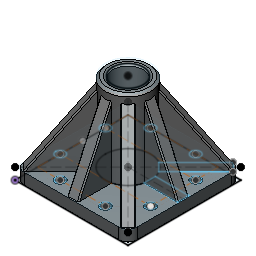
Кронштейн под лампу v1 (Autodesk Fusion 360 design; units mm, degrees)
Autodesk Fusion 360 part; units mm, degrees
sketch "Sketch1" plane through (0, 0, 0) normal (0, 0, 1) x (1, 0, 0)
  line L0 (0, 0) -> (50, 0)
  line L1 (50, 0) -> (50, 50)
  line L2 (50, 50) -> (0, 50)
  line L3 (0, 50) -> (0, 0)
  dimension "d1" = 50
  dimension "d2" = 50
  constraint horizontal L0
  constraint vertical L1
  constraint horizontal L2
  constraint vertical L3
  constraint coincident L0.start L3.end
  measures "d1" distance of L0.start L0.end
  measures "d2" distance of L0.start L2.end
extrude "Extrude1" add sketch "Sketch1" along normal blind 5 makes body 1
sketch "Sketch2" plane through (0, 0, 5) normal (0, 0, 1) x (-1, 0, 0)
  line L0 (0, -50) -> (0, 0)
  line L1 (0, 0) -> (-50, 0)
  line L2 (-50, 0) -> (-50, -50)
  line L3 (-50, -50) -> (0, -50)
  circle A0 centre (-25, -25) radius 10
  line L4 (0, -50) -> (-50, 0) construction
  line L5 (-50, -50) -> (0, 0) construction
  line L6 (-25, -25) -> (-50, -25) construction
  line L7 (-34.6825, -22.5) -> (-49.4483, -22.5)
  line L8 (-49.4483, -22.5) -> (-49.4483, -27.5)
  line L9 (-34.6825, -27.5) -> (-49.4483, -27.5)
  line L10 (-34.6825, -27.5) -> (-34.6825, -22.5)
  line L11 (-50, -46.4645) -> (-46.4645, -50)
  line L12 (-46.4645, -50) -> (-30.0788, -33.6143)
  line L13 (-30.0788, -33.6143) -> (-33.6143, -30.0788)
  line L14 (-33.6143, -30.0788) -> (-50, -46.4645)
  line L15 (-45, -35) -> (-45, -45) construction
  line L16 (-45, -45) -> (-35, -45) construction
  line L17 (-35, -45) -> (-25, -45) construction
  line L18 (-25, -45) -> (-15, -45) construction
  line L19 (-15, -45) -> (-5, -45) construction
  line L20 (-5, -45) -> (-5, -35) construction
  line L21 (-5, -35) -> (-45, -35) construction
  line L22 (-45, -35) -> (-45, -15) construction
  line L23 (-45, -15) -> (-5, -15) construction
  line L24 (-5, -15) -> (-5, -25) construction
  line L25 (-5, -15) -> (-5, -5) construction
  line L26 (-5, -5) -> (-15, -5) construction
  line L27 (-15, -5) -> (-35, -5) construction
  circle A1 centre (-45, -35) radius 2
  circle A2 centre (-45, -15) radius 2
  circle A3 centre (-5, -35) radius 2
  circle A4 centre (-35, -45) radius 2
  circle A5 centre (-15, -45) radius 2
  circle A6 centre (-5, -15) radius 2
  circle A7 centre (-15, -5) radius 2
  circle A8 centre (-35, -5) radius 2
  dimension "d5" = 20
  dimension "d18" = 5
  dimension "d32" = 10
  dimension "d33" = 10
  dimension "d34" = 10
  dimension "d35" = 10
  dimension "d36" = 4
  dimension "d43" = 4
  dimension "d44" = 4
  dimension "d45" = 4
  dimension "d46" = 4
  dimension "d47" = 4
  dimension "d48" = 4
  dimension "d49" = 4
  constraint coincident L0.start L3.end
  constraint coincident L1.end L2.start
  constraint coincident L2.end L3.start
  constraint coincident L0.end L1.start
  constraint midpoint A0.centre L5
  constraint coincident A0.centre L6.start
  constraint midpoint L2 L6.end
  constraint perpendicular L6 L8
  constraint coincident A0 L9.start
  constraint perpendicular L8 L9
  constraint coincident A0 L7.start
  constraint horizontal L7
  constraint coincident L2 L11.start
  constraint coincident L3 L11.end
  constraint coincident A0 L12.end
  constraint perpendicular L11 L12
  constraint coincident A0 L13.end
  constraint perpendicular L5 L13
  constraint perpendicular L11 L14
  constraint coincident L5 L15.end
  constraint vertical L15
  constraint perpendicular L15 L16
  constraint parallel L16 L17
  constraint parallel L17 L18
  constraint coincident L4 L19.end
  constraint perpendicular L0 L19
  constraint perpendicular L19 L20
  constraint perpendicular L15 L21
  constraint perpendicular L7 L22
  constraint perpendicular L22 L23
  constraint perpendicular L21 L24
  constraint perpendicular L23 L25
  constraint perpendicular L25 L26
  constraint perpendicular L25 L27
  constraint coincident L15.start L21.end
  constraint coincident L16.end L17.start
  constraint coincident L18.end L19.start
  constraint coincident L23.end L24.start
  constraint coincident L26.end L27.start
  constraint coincident L27.end A8.centre
  measures "d5" diameter of A0
  measures "d18" distance of L7.end L8.end
  measures "d32" distance of L15.end L16.end
  measures "d33" distance of L17.end L18.end
  measures "d34" distance of L23.end L25.end
  measures "d35" distance of L25.end L26.end
  measures "d36" diameter of A1
  measures "d43" diameter of A2
  measures "d44" diameter of A3
  measures "d45" diameter of A4
  measures "d46" diameter of A5
  measures "d47" diameter of A6
  measures "d48" diameter of A7
  measures "d49" diameter of A8
extrude "Extrude2" add sketch "Sketch2" along normal blind 35 contours A0 L10 L13 | A0 L13 | A0 L10 bodies 1
sketch "Sketch3" plane through (0, 0, 40) normal (0, 0, 1) x (-1, 0, 0)
  circle A0 centre (-25, -25) radius 10
  circle A1 centre (-25, -25) radius 6.75
  dimension "d8" = 13.5
  constraint concentric A0 A1
  measures "d8" diameter of A1
extrude "Extrude3" cut sketch "Sketch3" against normal blind 40 contours A1 bodies 1
extrude "Extrude4" add sketch "Sketch2" along normal blind 33 separate body contours A0 L7 L8 L9 makes body 2
extrude "Extrude5" add sketch "Sketch2" along normal blind 33 separate body contours A0 L11 L12 L14 makes body 3
draft "Draft1" angle 25 neutral plane through (0, 0, 5) pull (0, 0, 1) 1 faces at (49.4483, 24.1667, 16) on bodies 2
draft "Draft2" angle 36.3 neutral plane through (0, 0, 5) pull (0, 0, 1) 1 faces at (47.643, 48.8215, 27) on bodies 3
pattern_circular "C-Pattern1" count 4 over 360 about axis through (25, 25, 5) along (0, 0, 1) of bodies 2 makes body 4 at (22.5, 39.6044, 15.5552) makes body 5 at (10.3956, 22.5, 15.5552) makes body 6 at (27.5, 10.3956, 15.5552)
pattern_circular "C-Pattern2" count 4 over 360 about axis through (25, 25, 5) along (0, 0, 1) of bodies 3 makes body 7 at (14.4593, 39.0762, 15.5154) makes body 8 at (10.9238, 14.4593, 15.5154) makes body 9 at (35.5407, 10.9238, 15.5154)
extrude "Extrude9" cut sketch "Sketch2" against normal blind 5 contours A1 | A2 | A3 | A4 | A5 | A6 | A7 | A8 bodies 1
chamfer "Chamfer1" distance 1 angle 45 1 edges at (31.2932, 22.5591, 40) on bodies 1
chamfer "Chamfer2" distance 1 angle 45 1 edges at (34.3233, 28.6162, 40) on bodies 1
chamfer "Chamfer3" distance 0.5 angle 45 16 edges at (22.5, 42.0654, 20.8327) (27.5, 42.0654, 20.8327) (38.2716, 41.8071, 20.773) (41.8071, 38.2716, 20.773) (11.7284, 8.1929, 20.773) (8.1929, 11.7284, 20.773) (41.8071, 11.7284, 20.773) (38.2716, 8.1929, 20.773) (8.1929, 38.2716, 20.773) (11.7284, 41.8071, 20.773) (42.0654, 22.5, 20.8327) (42.0654, 27.5, 20.8327) (7.9346, 22.5, 20.8327) (7.9346, 27.5, 20.8327) (27.5, 7.9346, 20.8327) (22.5, 7.9346, 20.8327) on bodies 2 3 4 5 6 7 8 9
fillet "Fillet1" radius 4 1 edges at (50, 0, 2.5) on bodies 1
fillet "Fillet2" radius 4 3 edges at (0, 0, 2.5) (0, 50, 2.5) (50, 50, 2.5) on bodies 1
fillet "Fillet3" radius 0.1 8 edges at (25, 50, 0) (1.1716, 48.8284, 0) (0, 25, 0) (1.1716, 1.1716, 0) (25, 0, 0) (48.8284, 1.1716, 0) (50, 25, 0) (48.8284, 48.8284, 0) on bodies 1
chamfer "Chamfer4" distance 0.2 angle 45 8 edges at (6.8647, 34.2768, 5) (16.8647, 44.2768, 5) (6.8647, 14.2768, 5) (16.8647, 4.2768, 5) (36.8647, 44.2768, 5) (46.8647, 34.2768, 5) (46.8647, 14.2768, 5) (36.8647, 4.2768, 5) on bodies 1
